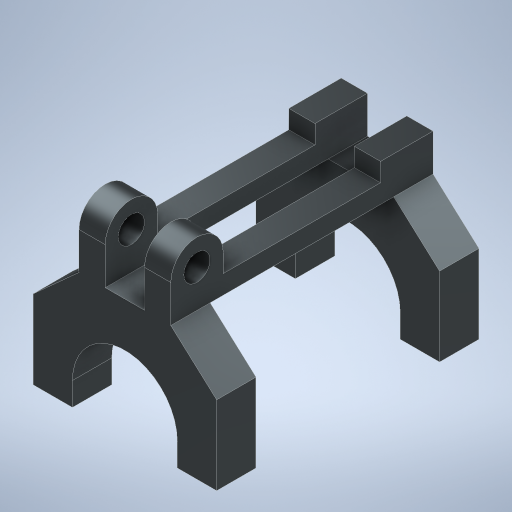
# Autodesk Inventor part: ASN4-4-BK
Saved by Autodesk Inventor 2024 (Build 280153000, 153)
## iProperties
Created: 2023-09-23
Part Number: ASN4-4-BK
Material: Iron, Cast
Document SubType Name: Modeling
Designer: bennk
Density: 7.15 g/cm^3
Appearance: Iron Gray
Author: bennk
Autodesk Inventor part; units mm, degrees
ref_plane "YZ Plane" through (0, 0, 0) normal (1, 0, 0) x (0, 1, 0)
ref_plane "XZ Plane" through (0, 0, 0) normal (0, 1, 0) x (-1, 0, 0)
ref_plane "XY Plane" through (0, 0, 0) normal (0, 0, 1) x (1, 0, 0)
sketch "front profile" plane through (0, 0, 0) normal (0, 0, 1) x (1, 0, 0)
  line L0 (47.7209, 56.8325) -> (47.7209, 18.7325)
  line L1 (-41.1791, 18.7325) -> (-41.1791, 56.8325)
  line L2 (25.4959, 107.6325) -> (25.4959, 76.9011)
  line L3 (12.7959, 76.9011) -> (-6.2541, 76.9011)
  line L4 (-18.9541, 76.9011) -> (-18.9541, 107.6325)
  line L5 (12.7959, 107.6325) -> (12.7959, 76.9011)
  line L6 (12.7959, 76.9011) -> (-6.2541, 76.9011)
  line L7 (-6.2541, 76.9011) -> (-6.2541, 107.6325)
  line L8 (25.4959, 76.9011) -> (47.7209, 56.8325)
  line L9 (-18.9541, 76.9011) -> (-41.1791, 56.8325)
  line L10 (28.6709, 18.7325) -> (28.6709, 30.003)
  line L11 (-22.1291, 30.003) -> (-22.1291, 18.7325)
  arc A0 (28.6709, 30.003) -> (-22.1291, 30.003) centre (3.2709, 30.003) ccw
  line L12 (-18.9541, 107.6325) -> (-6.2541, 107.6325)
  line L13 (12.7959, 107.6325) -> (25.4959, 107.6325)
  line L14 (47.7209, 18.7325) -> (28.6709, 18.7325)
  line L15 (-22.1291, 18.7325) -> (-41.1791, 18.7325)
  line L16 (-18.9541, 107.6325) -> (-6.2541, 107.6325)
  line L17 (12.7959, 107.6325) -> (25.4959, 107.6325)
  point P0 (0, 0)
  point P1 (-6.2541, 92.2668)
  point P2 (-12.6041, 107.6325)
  point P3 (19.1459, 107.6325)
  dimension "d2" = 88.9
  dimension "d9" = 22.225
  dimension "d10" = 22.225
  dimension "d11" = 12.7
  dimension "d12" = 12.7
  dimension "d14" = 38.1
  dimension "d15" = 38.1
  dimension "d17" = 19.05
  dimension "d18" = 19.05
  dimension "d32" = 88.9
  dimension "d33" = 88.9
  dimension "d34" = 25.4
  dimension "d36" = 47.919
  dimension "d37" = 47.919
  dimension "d39" = 58.1686
  constraints: 36 end point, 10 parallel, 4 horizontal, 4 perpendicular, 3 midpoint, 2 point on circle, 2 tangent, 1 centre point
  measures "d2" distance between parallel lines of L0 L1
  measures "d9" distance between parallel lines of L0 L2
  measures "d10" distance between parallel lines of L1 L4
  measures "d11" distance between parallel lines of L2 L5
  measures "d12" distance from line of L4 point (-6.254, 92.267)
  measures "d14" distance of L0.start L0.end
  measures "d15" distance of L1.end L1.start
  measures "d17" distance of L10.start L0.end
  measures "d18" distance of L11.end L1.start
  measures "d32" distance from line of point (-12.604, 107.632) L15
  measures "d33" distance from line of point (19.146, 107.632) L14
  measures "d34" radius of A0
  measures "d36" angle of L0 L8
  measures "d37" angle of L1 L9
  measures "d39" distance between parallel lines of L3 L14
extrude "front profile Extrusion" add sketch "front profile" along normal blind 127
sketch "side profile" plane through (25.4959, 76.9011, 0) normal (1, 0, 0) x (0, 0, -1)
  line L0 (0, -20.0686) -> (0, -58.1686) projected
  line L1 (-127, 30.7314) -> (0, 30.7314)
  line L2 (0, 30.7314) -> (0, -58.1686)
  line L3 (0, -58.1686) -> (-127, -58.1686)
  line L4 (-127, -58.1686) -> (-127, 18.0314)
  line L5 (-25.4, 18.0314) -> (-25.4, 9.0465)
  line L6 (-25.4, 9.0465) -> (-101.6, 9.0465)
  line L7 (-101.6, 9.0465) -> (-101.6, 18.0314)
  line L8 (0, 0) -> (-127, 0) projected
  line L9 (0, -58.1686) -> (-127, -58.1686) projected
  line L10 (-107.95, 0) -> (-19.05, 0)
  line L11 (-19.05, 0) -> (-19.05, -58.1686)
  line L12 (-19.05, -58.1686) -> (-107.95, -58.1686)
  line L13 (-107.95, -58.1686) -> (-107.95, 0)
  circle A0 centre (-114.3, 18.0314) radius 6.35
  arc A1 (-101.6, 18.0314) -> (-127, 18.0314) centre (-114.3, 18.0314) ccw
  line L14 (0, 30.7314) -> (-127, 30.7314) projected
  line L15 (-25.4, 18.0314) -> (0, 18.0314)
  point P0 (0, -76.9011)
  point P1 (-114.3, 30.7314)
  point P2 (-107.95, -58.1686)
  point P3 (-19.05, -58.1686)
  point P4 (-19.05, 0)
  dimension "d23" = 25.4
  dimension "d24" = 19.05
  dimension "d25" = 19.05
  dimension "d26" = 12.7
  dimension "d27" = 12.7
  dimension "d35" = 127
  constraints: 24 end point, 5 parallel, 3 horizontal, 3 point on line, 3 tangent, 2 centre point, 2 perpendicular, 2 point on circle
  measures "d23" distance between parallel lines of L2 L5
  measures "d24" distance between parallel lines of L0 L11
  measures "d25" distance between parallel lines of L4 L13
  measures "d26" diameter of A0
  measures "d27" distance from line of L4 A0.centre
  measures "d35" distance of L0.end L3.end
extrude "side profile extrusion" cut sketch "side profile" along normal through all both and the other way through all contours L3 L13 L8 L11 | L15 L5 L6 L7 A1 L1 L2 | A0
fillet "Front Fillet" radius 12.7 2 edges at (19.1459, 107.6325, 127) (-12.6041, 107.6325, 127)
equation "\"d10\" = d9"
equation "\"d12\" = d11"
equation "\"d15\" = d14"
equation "\"d17\" = d16"
equation "\"d33\" = d32"
equation "\"d37\" = d36"
equation "\"d25\" = d24"
equation "\"d16\" = 19.05"
body "Solid1"
